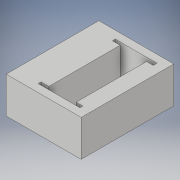
# Autodesk Inventor part: hole
Saved by Autodesk Inventor 2019.3 (Build 233278000, 278)
## iProperties
Created: 2019-05-30
Part Number: hole
Material: Generic
Document SubType Name: Modeling
Designer: Frienddo
Density: 1 g/cm^3
Appearance: Default
Author: Frienddo
Autodesk Inventor part; units mm, degrees
ref_plane "YZ Plane" through (0, 0, 0) normal (1, 0, 0) x (0, 1, 0)
ref_plane "XZ Plane" through (0, 0, 0) normal (0, 1, 0) x (-1, 0, 0)
ref_plane "XY Plane" through (0, 0, 0) normal (0, 0, 1) x (1, 0, 0)
sketch "Sketch1" plane through (0, 0, 0) normal (0, 1, 0) x (-1, 0, 0)
  line L0 (-15.5, -19.25) -> (15.5, -19.25)
  line L1 (15.5, -19.25) -> (15.5, 19.25)
  line L2 (15.5, 19.25) -> (-15.5, 19.25)
  line L3 (-15.5, 19.25) -> (-15.5, -19.25)
  line L4 (-15.5, -19.25) -> (15.5, 19.25) construction
  line L5 (15.5, -19.25) -> (-15.5, 19.25) construction
  line L6 (2.75, 0) -> (2.75, 14.75)
  line L7 (2.75, 14.75) -> (6, 14.75)
  line L8 (6, 14.75) -> (6, 16.75)
  line L9 (6, 16.75) -> (-3.25, 16.75)
  line L10 (-3.25, 16.75) -> (-3.25, 0)
  line L11 (-3.25, 0) -> (2.75, 0)
  line L12 (2.75, 0) -> (2.75, -14.75)
  line L13 (2.75, -14.75) -> (6, -14.75)
  line L14 (6, -14.75) -> (6, -16.75)
  line L15 (6, -16.75) -> (-3.25, -16.75)
  line L16 (-3.25, -16.75) -> (-3.25, 0)
  line L17 (-9.25, 0) -> (-9.25, 14.75)
  line L18 (-9.25, 14.75) -> (-12.5, 14.75)
  line L19 (-12.5, 14.75) -> (-12.5, 16.75)
  line L20 (-12.5, 16.75) -> (-3.25, 16.75)
  line L21 (-12.5, -14.75) -> (-12.5, -16.75)
  line L22 (-9.25, -14.75) -> (-12.5, -14.75)
  line L23 (-9.25, 0) -> (-9.25, -14.75)
  line L24 (-12.5, -16.75) -> (-3.25, -16.75)
  point P0 (0, 0)
  dimension "d0" = 31
  dimension "d1" = 38.5
  dimension "d2" = 2
  dimension "d3" = 2.5
  dimension "d4" = 2.5
  dimension "d5" = 3
  dimension "d6" = 18.5
  dimension "d7" = 12
  constraints: 50 end point, 11 symmetric about line, 5 perpendicular, 2 horizontal, 2 midpoint, 2 parallel, 1 vertical
  measures "d0" distance of L2.end L1.end
  measures "d1" distance of L0.end L1.end
  measures "d2" distance of L7.end L8.end
  measures "d3" distance between parallel lines of L2 L9
  measures "d4" distance between parallel lines of L0 L15
  measures "d5" distance between parallel lines of L3 L19
  measures "d6" distance between parallel lines of L19 L8
  measures "d7" distance between parallel lines of L17 L6
extrude "Extrusion1" add sketch "Sketch1" along normal blind 15
thicken "Thicken1" operation add thickness 0.4 both sides no extend neighbours yes toward (1, 0, 0) faces at (-2.75, 10, -9.8333) (-2.75, 10, 4.9167) (-3.8333, 5, 14.75) (-6, 5, 15.4167) (-2.9167, 5, 16.75) (6.3333, 10, 16.75) (-11.25, 0, 0) (11.4167, 5, 14.75) (12.5, 5, 16.0833) (-4.9167, 5, -14.75) (9.4167, 5, -16.75) (0.1667, 10, -16.75) (-6, 5, -16.0833) (12.5, 5, -15.4167)
thicken "Thicken2" operation add thickness 0.4 both sides no extend neighbours yes toward (0, 0, 1) faces at (5.1667, 9.8667, 19.25) (15.5, 9.8667, 6.4167) (-15.5, 9.8667, 6.4167) (5.1667, 4.7333, -19.25)
body "Solid1"
